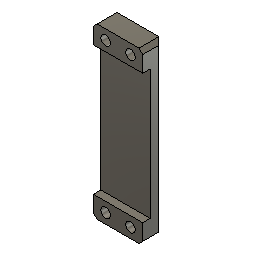
_Platform Link Arm.c20c3072-6dc2-4d8d-a4cd-072d7f1dbc6d (Autodesk Fusion 360 design; units mm, degrees)
Autodesk Fusion 360 part; units mm, degrees
sketch "Sketch1" plane through (0, 0, 0) normal (0, 0, 1) x (1, 0, 0)
  line L0 (0, 0) -> (19.8, 0)
  line L1 (19.8, 0) -> (19.8, 34)
  line L2 (19.8, 34) -> (0, 34)
  circle A0 centre (14.9, 4) radius 1.9
  circle A1 centre (4.9, 4) radius 1.9
  line L3 (14.9, 1) -> (19.8, 1)
  line L4 (4.9, 1) -> (0, 1)
  line L5 (19.8, 1) -> (19.8, 0)
  line L6 (0, 0) -> (0, 1)
  line L7 (0, 0) -> (0, 34)
  circle A2 centre (4.9, 4) radius 3
  circle A3 centre (14.9, 4) radius 3
  line L8 (0, 8) -> (19.8, 8)
  line L9 (19.8, 8) -> (19.8, 0)
  line L10 (19.8, 4) -> (21.7184, 4)
  line L11 (14.9, 4) -> (15.5, 4)
  line L12 (4.9, 4) -> (6, 4)
  line L13 (9.9, 0) -> (9.9, 34)
  dimension "d1" = 10
  dimension "d3" = 3.8
  dimension "d5" = 4.9
  dimension "d7" = 6
  dimension "d9" = 30
  dimension "d10" = 8
  constraint horizontal L0
  constraint vertical L1
  constraint horizontal L2
  constraint coincident L0.start L6.start
  constraint equal A0 A1
  constraint coincident L1 L3.end
  constraint equal L3 L4
  constraint horizontal L4
  constraint equal L5 L6
  constraint perpendicular L4 L6
  constraint perpendicular L0 L7
  constraint concentric A1 A2
  constraint concentric A0 A3
  constraint tangent L3 A3
  constraint tangent L4 A2
  constraint coincident L4.start A2
  constraint coincident L3.start A3
  constraint equal A2 A3
  constraint coincident L7 L8.start
  constraint coincident L1 L8.end
  constraint perpendicular L1 L8
  constraint perpendicular L1 L3
  constraint midpoint L9 L10.start
  constraint perpendicular L1 L10
  constraint coincident A0.centre A3.centre
  constraint parallel L8 L11
  constraint coincident A1.centre A2.centre
  constraint parallel L8 L12
  constraint collinear L10 L11
  constraint midpoint L0 L13.start
  constraint midpoint L2 L13.end
  measures "d1" distance of A0.centre A1.centre
  measures "d3" diameter of A1
  measures "d5" distance of L4.start L4.end
  measures "d7" diameter of A2
  measures "d9" distance of L2 A1.centre
  measures "d10" distance of L0 L8
extrude "Extrude1" add sketch "Sketch1" along normal blind 8 contours L0 L1 L5 L8 L9 L13
extrude "Extrude2" add sketch "Sketch1" along normal blind 5 contours L1 L2 L8 L13
extrude "Extrude3" add sketch "Sketch1" along normal blind 8 and the other way blind -5 contours A3
chamfer "Chamfer1" distance 1.5 angle 45 2 edges at (19.8, 17, 0) (19.8, 0, 4)
mirror "Mirror1" about plane through (19.8, 34, 0) normal (0, 1, 0) of bodies 1 merged
mirror "Mirror2" about plane through (9.9, 0, 0) normal (-1, 0, 0) of bodies 1 merged
equation "d5 = ( 3.8 / 2 ) * 1 mm + 3 mm"
equation "d17 = -8.00 mm + 3 mm"
named bodies: "Link Arm Platform"
